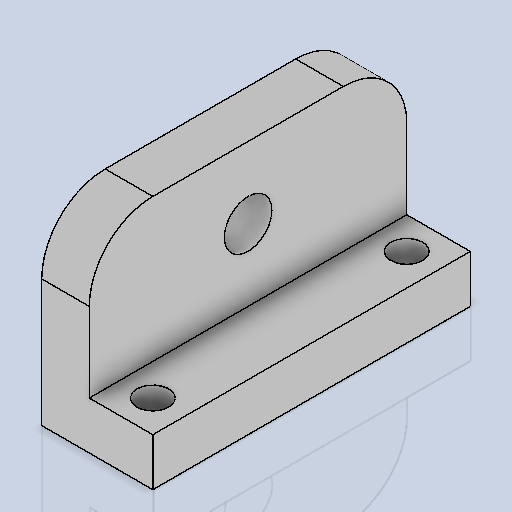
# Autodesk Inventor part: drum_holder
Saved by Autodesk Inventor 2026.1 (Build 301233000, 233)
## iProperties
Created: 2025-08-31
Part Number: drum_holder
Material: Generic
Document SubType Name: Modeling
Designer: baseb
Density: 1 g/cm^3
Appearance: Default
Author: baseb
Autodesk Inventor part; units mm, degrees
ref_plane "YZ Plane" through (0, 0, 0) normal (1, 0, 0) x (0, 1, 0)
ref_plane "XZ Plane" through (0, 0, 0) normal (0, 1, 0) x (-1, 0, 0)
ref_plane "XY Plane" through (0, 0, 0) normal (0, 0, 1) x (1, 0, 0)
sketch "Sketch1" plane through (0, 0, 0) normal (0, 1, 0) x (-1, 0, 0)
  line L0 (-6.35, 31.75) -> (6.35, 31.75)
  line L1 (6.35, 31.75) -> (6.35, -31.75)
  line L2 (6.35, -31.75) -> (-6.35, -31.75)
  line L3 (-6.35, -31.75) -> (-6.35, 31.75)
  line L4 (-6.35, 31.75) -> (6.35, -31.75) construction
  line L5 (6.35, 31.75) -> (-6.35, -31.75) construction
  circle A0 centre (0, 25.4) radius 3.175
  circle A1 centre (0, -25.4) radius 3.175
  point P0 (0, 0)
  dimension "d0" = 12.7
  dimension "d1" = 63.5
  dimension "d2" = 6.35
  dimension "d3" = 6.35
  dimension "d4" = 50.8
  dimension "d5" = 6.35
  constraints: 12 end point, 2 centre point, 2 midpoint, 2 parallel, 1 horizontal, 1 perpendicular
  measures "d0" distance of L1.end L2.end
  measures "d1" distance of L0.end L1.end
  measures "d2" diameter of A0
  measures "d3" diameter of A1
  measures "d4" distance of A1.centre A0.centre
  measures "d5" distance from line of L0 A0.centre
extrude "Extrusion1" add sketch "Sketch1" along normal blind 9.525
sketch "Sketch2" plane through (0, 0, 0) normal (0, 1, 0) x (-1, 0, 0)
  line L0 (6.35, -31.75) -> (6.35, 31.75) projected
  line L1 (6.35, 31.75) -> (15.875, 31.75)
  line L2 (15.875, 31.75) -> (15.875, -31.75)
  line L3 (15.875, -31.75) -> (6.35, -31.75)
  line L4 (6.35, -31.75) -> (6.35, 31.75)
  point P0 (0, 0)
  dimension "d8" = 9.525
  constraints: 8 end point, 2 parallel, 1 horizontal, 1 perpendicular
  measures "d8" distance of L2.end L3.end
extrude "Extrusion2" add sketch "Sketch2" along normal blind 38.1
fillet "Fillet1" radius 12.7 2 edges at (-11.1125, 38.1, 31.75) (-11.1125, 38.1, -31.75)
sketch "Sketch3" plane through (-15.875, 0, -31.75) normal (-1, 0, 0) x (0, 0, 1)
  line L0 (50.8, 38.1) -> (12.7, 38.1) projected
  line L1 (31.75, 38.1) -> (31.75, 23.8125) construction
  circle A0 centre (31.75, 23.8125) radius 4.7625
  point P0 (31.75, 0)
  dimension "d12" = 14.2875
  dimension "d13" = 9.525
  constraints: 2 end point, 1 centre point, 1 coincident, 1 midpoint, 1 vertical
  measures "d12" distance of L1.start L1.end
  measures "d13" diameter of A0
extrude "Extrusion3" cut sketch "Sketch3" against normal through all
equation "\"d3\" = d2"
body "Solid1"
